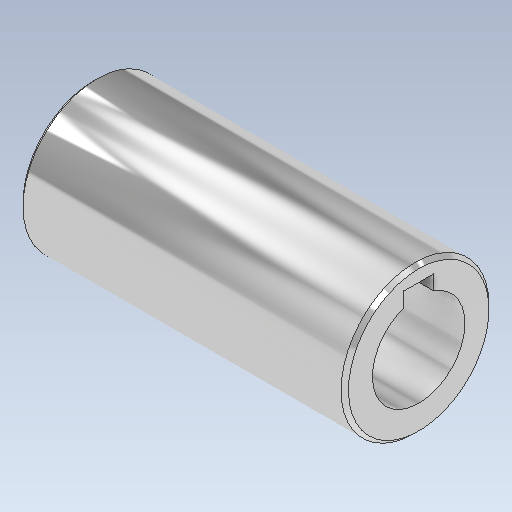
# Autodesk Inventor part: outputshaft nmrv50
Saved by Autodesk Inventor 2020 (Build 240168000, 168)
## iProperties
Created: 2020-07-31
Part Number: outputshaft nmrv50
Material: Generic
Document SubType Name: Modeling
Designer: Vikki
Density: 1 g/cm^3
Appearance: Chrome - Polished
Mass: 64.7878 g
Surface Area: 199.792 cm^2
Volume: 64.7878 cm^3
Author: Vikki
Autodesk Inventor part; units mm, degrees
ref_plane "YZ Plane" through (0, 0, 0) normal (1, 0, 0) x (0, 1, 0)
ref_plane "XZ Plane" through (0, 0, 0) normal (0, 1, 0) x (-1, 0, 0)
ref_plane "XY Plane" through (0, 0, 0) normal (0, 0, 1) x (1, 0, 0)
sketch "Sketch1" plane through (0, 0, 0) normal (1, 0, 0) x (0, 1, 0)
  circle A0 centre (0, 0) radius 20
  circle A1 centre (0, 0) radius 12.5
  line L0 (15.8, 4) -> (15.8, -4)
  line L1 (15.8, 4) -> (11.8427, 4)
  line L2 (15.8, -4) -> (11.8427, -4)
  dimension "d0" = 40
  dimension "d1" = 25
  dimension "d2" = 8
  dimension "d3" = 4
  dimension "d4" = 15.8
  constraints: 6 end point, 2 centre point, 2 coincident, 2 horizontal, 2 point on circle, 1 vertical
  measures "d0" diameter of A0
  measures "d1" diameter of A1
  measures "d2" distance of L0.start L0.end
  measures "d3" vertical distance of point (0, 0) L0.start
  measures "d4" distance from line of point (0, 0) L0
extrude "Extrusion1" add sketch "Sketch1" along normal blind 88
chamfer "Chamfer1" distance 1 angle 45 2 edges at (88, -20, 0) (0, -20, 0)
body "Solid1"
